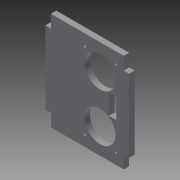
# Autodesk Inventor part: faceplate_ultrasound
Saved by Autodesk Inventor 2015 SP2 (Build 190223200, 223)
## iProperties
Created: 2015-11-14
Part Number: faceplate_ultrasound
Material: Generic
Document SubType Name: Modeling
Designer: styku
Density: 1 g/cm^3
Appearance: Default
Author: styku
Autodesk Inventor part; units mm, degrees
ref_plane "YZ Plane" through (0, 0, 0) normal (1, 0, 0) x (0, 1, 0)
ref_plane "XZ Plane" through (0, 0, 0) normal (0, 1, 0) x (-1, 0, 0)
ref_plane "XY Plane" through (0, 0, 0) normal (0, 0, 1) x (1, 0, 0)
sketch "Sketch1" plane through (0, 0, 0) normal (0, 1, 0) x (-1, 0, 0)
  line L0 (38.75, 0) -> (-38.75, 0) construction
  line L1 (0, 44.6319) -> (0, -56.6181) construction
  line L2 (0, 27) -> (20, 27)
  line L3 (20, 27) -> (20, 20)
  line L4 (20, 20) -> (23, 20)
  line L5 (23, 20) -> (23, 0)
  line L6 (0, -27) -> (20, -27)
  line L7 (20, -27) -> (20, -20)
  line L8 (20, -20) -> (23, -20)
  line L9 (23, -20) -> (23, 0)
  line L10 (0, 27) -> (-20, 27)
  line L11 (-20, 27) -> (-20, 20)
  line L12 (-20, 20) -> (-23, 20)
  line L13 (-23, 20) -> (-23, 0)
  line L14 (0, -27) -> (-20, -27)
  line L15 (-20, -27) -> (-20, -20)
  line L16 (-23, -20) -> (-23, 0)
  line L17 (-20, -20) -> (-23, -20)
  line L18 (3, 22.5) -> (-17, 22.5) construction
  line L19 (-17, 22.5) -> (-17, -22.5) construction
  line L20 (-17, -22.5) -> (3, -22.5) construction
  line L21 (3, -22.5) -> (3, 22.5) construction
  line L22 (19.5, 12.5) -> (-4.5, 12.5) construction
  line L23 (-4.5, 12.5) -> (-4.5, -12.5) construction
  line L24 (-4.5, -12.5) -> (19.5, -12.5) construction
  line L25 (19.5, -12.5) -> (19.5, 12.5) construction
  circle A0 centre (-7, 13) radius 8.5
  circle A1 centre (-7, -13) radius 8.5
  circle A2 centre (1.5, 21) radius 0.75
  circle A3 centre (1.5, -21) radius 0.75
  line L26 (-7, 17.5) -> (-7, -18.0475) construction
  circle A4 centre (-15.5, 21) radius 0.75
  circle A5 centre (-15.5, -21) radius 0.75
  line L27 (-16, 5.5) -> (-12, 5.5)
  line L28 (-12, 5.5) -> (-12, -5.5)
  line L29 (-12, -5.5) -> (-16, -5.5)
  line L30 (-16, -5.5) -> (-16, 5.5)
  point P0 (0, 0)
  point P1 (0, 0)
  dimension "d0" = 20
  dimension "d1" = 27
  dimension "d3" = 20
  dimension "d4" = 20
  dimension "d5" = 45
  dimension "d7" = 24
  dimension "d8" = 25
  dimension "d9" = 0.5
  dimension "d10" = 17
  dimension "d11" = 13
  dimension "d12" = 10
  dimension "d13" = 1.5
  dimension "d14" = 1.5
  dimension "d15" = 1.5
  dimension "d16" = 3
  dimension "d30" = 3
  dimension "d31" = 4
  dimension "d32" = 11
  dimension "d33" = 1
  constraints: 62 end point, 15 symmetric about line, 6 centre point, 6 parallel, 6 perpendicular, 5 horizontal, 4 point on line, 2 vertical, 1 coincident, 1 midpoint, 7 other
  measures "d0" distance between parallel lines of L0 L4
  measures "d1" distance between parallel lines of L0 L2
  measures "d3" distance between parallel lines of L1 L3
  measures "d4" distance of L20.end L19.end
  measures "d5" distance of L19.end L18.end
  measures "d7" distance of L24.end L23.end
  measures "d8" distance of L23.end L22.end
  measures "d9" distance between parallel lines of L7 L25
  measures "d10" diameter of A0
  measures "d11" distance from line of L0 A0.centre
  measures "d12" distance from line of L21 A0.centre
  measures "d13" diameter of A2
  measures "d14" distance from line of L21 A2.centre
  measures "d15" distance from line of L18 A2.centre
  measures "d16" distance between parallel lines of L15 L19
  measures "d30" distance between parallel lines of L11 L13
  measures "d31" distance of L28.end L29.end
  measures "d32" distance of L27.end L28.end
  measures "d33" distance between parallel lines of L19 L30
extrude "Extrusion2" add sketch "Sketch1" along normal blind 3
body "Solid2"
